# Autodesk Inventor part: Flache Riemenscheibe1
Saved by Autodesk Inventor 2016 (Build 200138000, 138)
## iProperties
Created: 2015-08-10
Part Number: Flache Riemenscheibe1
Material: Steel
Document SubType Name: Modeling
Designer: 4ndreas
Density: 7.85 g/cm^3
Appearance: Steel
CustomPartVersion: 1
Author: 4ndreas
Autodesk Inventor part; units mm, degrees
ref_plane "YZ Plane" through (0, 0, 0) normal (1, 0, 0) x (0, 1, 0)
ref_plane "XZ Plane" through (0, 0, 0) normal (0, 1, 0) x (-1, 0, 0)
ref_plane "XY Plane" through (0, 0, 0) normal (0, 0, 1) x (1, 0, 0)
sketch "Hauptskizze" plane through (0, 0, 0) normal (0, 0, 1) x (1, 0, 0)
  circle A0 centre (0, 0) radius 6.5
  dimension "d0" = 13
  constraints: 1 centre point, 1 coincident
  measures "d0" diameter of A0
extrude "Riemenscheibe" add sketch "Hauptskizze" along normal mid plane 17.6
equation "\"d0\" = da_D"
equation "\"d1\" = da_B"
equation "\"da_D\" = 13"
equation "\"da_B\" = 17.6"
body "Solid1"
